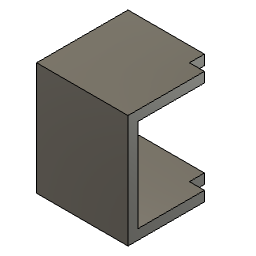
CORNER_CAP (Autodesk Fusion 360 design; units mm, degrees)
Autodesk Fusion 360 part; units mm, degrees
sketch "bottom" plane through (0, 0, 0) normal (0, 1, 0) x (1, 0, 0)
  circle A0 centre (0, 0) radius 2.5
  line L0 (12.5, -15) -> (-12.5, -15)
  line L1 (-12.5, -15) -> (-12.5, 15)
  line L2 (-12.5, 15) -> (12.5, 15)
  line L3 (12.5, 15) -> (12.5, -15)
  line L4 (12.5, -15) -> (-12.5, 15) construction
  line L5 (-12.5, -15) -> (12.5, 15) construction
  line L6 (-12.5, -15) -> (17.5, -15)
  line L7 (17.5, -15) -> (17.5, 10)
  line L8 (17.5, 10) -> (-12.5, 10)
  line L9 (-12.5, 10) -> (-12.5, -15)
  dimension "d1" = 5
  dimension "d2" = 25
  dimension "d3" = 30
  dimension "d4" = 30
  dimension "d5" = 25
  constraint coincident A0.centre origin
  constraint horizontal L0
  constraint perpendicular L0 L1
  constraint parallel L0 L2
  constraint parallel L1 L3
  constraint coincident L4 A0.centre
  constraint coincident L5 A0.centre
  constraint horizontal L6
  constraint vertical L7
  constraint horizontal L8
  constraint vertical L9
  measures "d1" diameter of A0
  measures "d2" distance of L1.end L2.end
  measures "d3" distance of L0.end L1.end
  measures "d4" distance of L0.end L6.end
  measures "d5" distance of L0.end L8.end
extrude "Extrude1" add sketch "bottom" along normal blind 3.352 makes body 1
sketch "Sketch2" plane through (0, 3.352, 0) normal (0, 1, 0) x (-1, 0, 0)
  circle A0 centre (0, 0) radius 2.5
  line L0 (12.5, -15) -> (12.5, 15)
  line L1 (12.5, 15) -> (-17.5, 15)
  line L2 (-17.5, 15) -> (-17.5, -10)
  line L3 (-17.5, -10) -> (-12.5, -10)
  line L4 (-12.5, -10) -> (-12.5, -15)
  line L5 (-12.5, -15) -> (12.5, -15)
  circle A1 centre (0, 0) radius 5
  dimension "d8" = 10
  constraint coincident A0.centre A1.centre
  measures "d8" diameter of A1
extrude "Extrude2" cut sketch "Sketch2" against normal blind 2 contours A1 bodies 1
ref_plane "WorkPlane1" through (2.5, 33.352, 0) normal (0, 1, 0) x (1, 0, 0)
sketch "Sketch3" plane through (0, 33.352, 0) normal (0, 1, 0) x (1, 0, 0)
  circle A0 centre (0, 0) radius 5
  line L0 (-12.5, 15) -> (-12.5, -15)
  line L1 (-12.5, -15) -> (17.5, -15)
  line L2 (17.5, -15) -> (17.5, 10)
  line L3 (17.5, 10) -> (12.5, 10)
  line L4 (12.5, 10) -> (12.5, 15)
  line L5 (12.5, 15) -> (-12.5, 15)
extrude "Extrude3" add sketch "Sketch3" along normal blind 3.352 separate body contours A0 | L0 L1 L2 L3 L4 L5 makes body 2
extrude "Extrude4" add 1 faces at (-4.1387, 1.352, -0.3726) along direction (0, 1, 0) blind 2 on bodies 1 bodies 1
sketch "Sketch4" plane through (0, 0, 0) normal (0, -1, 0) x (1, 0, 0)
  circle A0 centre (0, 0) radius 2.5
  line L0 (-12.5, 15) -> (-12.5, -15)
  line L1 (-12.5, -15) -> (12.5, -15)
  line L2 (12.5, -15) -> (12.5, -10)
  line L3 (12.5, -10) -> (17.5, -10)
  line L4 (17.5, -10) -> (17.5, 15)
  line L5 (17.5, 15) -> (-12.5, 15)
  circle A1 centre (0, 0) radius 5
  dimension "d16" = 10
  constraint coincident A0.centre A1.centre
  measures "d16" diameter of A1
extrude "Extrude5" cut sketch "Sketch4" against normal blind 2 contours A1 bodies 1
extrude "Extrude6" add 1 faces at (-4.1667, 36.704, -3.3333) along direction (0, 1, 0) blind 0.5 on bodies 2 bodies 2
extrude "Extrude7" cut 1 faces at (-4.1667, 33.352, -3.3333) along direction (0, 1, 0) blind 0.5 on bodies 2 bodies 2
extrude "Extrude8" add 2 faces at (-12.5, 34.9693, -5) (-12.5, 1.1173, 5) along direction (-1, 0, 0) blind 0.5 on bodies 1 2 bodies 2 1
extrude "Extrude9" add 2 faces at (-2.8333, 34.9693, 15) (7.3333, 2.2347, 15) along direction (0, 0, 1) blind 0.5 on bodies 1 2 bodies 2 1
sketch "Sketch5" plane through (0, 33.852, 0) normal (0, -1, 0) x (1, 0, 0)
  line L0 (-13, -15) -> (12.5, -15)
  line L1 (12.5, -15) -> (12.5, -10)
  line L2 (12.5, -10) -> (17.5, -10)
  line L3 (17.5, -10) -> (17.5, 15.5)
  line L4 (17.5, 15.5) -> (-13, 15.5)
  line L5 (-13, 15.5) -> (-13, -15)
  line L6 (-13, 15.5) -> (-9.648, 15.5)
  line L7 (-9.648, 15.5) -> (-9.648, -15)
  line L8 (-9.648, -15) -> (-13, -15)
  line L9 (-13, -15) -> (-13, 15.5)
  line L10 (-13, 15.5) -> (17.5, 15.5)
  line L11 (17.5, 15.5) -> (17.5, 12.148)
  line L12 (17.5, 12.148) -> (-13, 12.148)
  line L13 (-13, 12.148) -> (-13, 15.5)
  dimension "d27" = 3.352
  dimension "d28" = 30.5
  dimension "d29" = 3.352
  constraint horizontal L6
  constraint vertical L7
  constraint horizontal L8
  constraint vertical L9
  constraint coincident L4.end L5.start
  constraint horizontal L10
  constraint vertical L11
  constraint horizontal L12
  constraint vertical L13
  measures "d27" distance of L4.end L6.end
  measures "d28" distance of L4.end L0.start
  measures "d29" distance of L4.end L12.end
extrude "Extrude10" add sketch "Sketch5" along normal blind 30.5 contours L0 L5 L7 L8 L9 L12 | L4 L5 L6 L7 L9 L10 L12 L13 | L3 L4 L7 L10 L11 L12 bodies 1 2
extrude "Extrude11" add 1 faces at (1.0129, 3.352, -10.831) along direction (0, 1, 0) blind 0.5 on bodies 1 bodies 1
extrude "Extrude12" cut 1 faces at (13.3147, 0, 2.0817) along direction (0, 1, 0) blind 0.5 on bodies 1 bodies 1
extrude "Extrude13" add 1 faces at (4.1387, 2, -0.3726) along direction (0, -1, 0) blind 1.5 on bodies 1 bodies 1
extrude "Extrude14" add sketch "bottom" along normal blind 3.852 contours A0 bodies 1
extrude "Extrude15" cut 1 faces at (-0.8863, 0, -0.2321) along direction (0, 1, 0) blind 0.5 on bodies 1 bodies 1
extrude "Extrude16" cut 1 faces at (12.5, 34.9693, -11.6667) along direction (-1, 0, 0) blind 5 on bodies 1 bodies 1
extrude "Extrude17" cut 1 faces at (12.5, 1.6173, -13.3333) along direction (-1, 0, 0) blind 5 on bodies 1 bodies 1
extrude "Extrude18" cut 1 faces at (17.5, 23.852, 14.3827) along direction (-1, 0, 0) blind 5 on bodies 1 bodies 1
extrude "Extrude19" add 1 faces at (-11.8827, 23.852, -15) along direction (0, 0, -1) blind 5 on bodies 1 bodies 1
extrude "Extrude20" add 2 faces at (10.8333, 34.9693, -10) (10.8333, 1.6173, -10) along direction (0, 0, -1) blind 5 on bodies 1 bodies 1
extrude "Extrude21" add 1 faces at (2.3333, 0.5, 5.3333) along direction (0, -1, 0) blind 1 on bodies 1 bodies 1
extrude "Extrude22" cut 1 faces at (3.4507, 3.852, 3.0987) along direction (0, -1, 0) blind 1 on bodies 1 bodies 1
extrude "Extrude23" cut 2 faces at (9.1667, 1.7347, -15) (10.8333, 34.9693, -15) along direction (0, 0, 1) blind 5 on bodies 1 bodies 1
extrude "Extrude24" cut 1 faces at (-11.8827, 13.1853, -20) along direction (0, 0, 1) blind 5 on bodies 1 bodies 1
extrude "Extrude25" add 1 faces at (12.5, 23.5187, 14.3827) along direction (1, 0, 0) blind 5 on bodies 1 bodies 1
extrude "Extrude26" add 2 faces at (7.5, 36.0867, -11.6667) (7.5, 1.7347, -13.3333) along direction (1, 0, 0) blind 5 on bodies 1 bodies 1
